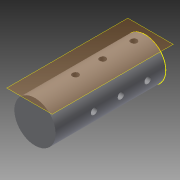
# Autodesk Inventor part: collector
Saved by Autodesk Inventor 2015 (Build 190159000, 159)
## iProperties
Created: 2014-11-05
Part Number: collector
Material: Generic
Document SubType Name: Modeling
Designer: lethcoec
Density: 1 g/cm^3
Appearance: Default
Author: lethcoec
Autodesk Inventor part; units mm, degrees
ref_plane "XY Plane" through (0, 0, 0) normal (0, 0, 1) x (1, 0, 0)
sketch "Sketch1" plane through (0, 0, 0) normal (0, 0, 1) x (1, 0, 0)
  circle A0 centre (0, 0) radius 19.05
  dimension "d0" = 38.1
  constraints: 1 centre point, 1 coincident
  measures "d0" diameter of A0
extrude "Extrusion1" add sketch "Sketch1" along normal blind 101.6
ref_plane "Work Plane1" through (19.05, 0, 0) normal (1, 0, 0) x (0, 1, 0)
sketch "Sketch3" plane through (19.05, 0, 0) normal (1, 0, 0) x (0, 1, 0)
  point P0 (0, 0)
sketch "Sketch4" plane through (19.05, 0, 0) normal (1, 0, 0) x (0, 1, 0)
  line L0 (0, 13.6144) -> (0, 19.5072)
  circle A0 centre (0, 16.5608) radius 2.9464
  point P0 (0, 0)
  dimension "d6" = 5.8928
  constraints: 2 end point, 1 midpoint, 1 vertical, 1 vertical alignment, 2 other
  measures "d6" distance of L0.start L0.end
hole "Hole1" at (19.05, 0, 16.5608) direction (-1, 0, 0) diameter 5.8928 end through all
sketch "Sketch5" plane through (19.05, 0, 0) normal (1, 0, 0) x (0, 1, 0)
  line L0 (0, 19.5072) -> (0, 38.354)
  line L1 (0, 38.354) -> (0, 44.2468)
  circle A0 centre (0, 41.3004) radius 2.9464
  point P0 (0, 0)
  dimension "d14" = 18.8468
  dimension "d15" = 5.8928
  constraints: 4 end point, 2 vertical, 1 midpoint, 1 vertical alignment, 2 other
  measures "d14" distance of L0.start L0.end
  measures "d15" distance of L0.end L1.end
hole "Hole2" at (19.05, 0, 41.3004) direction (-1, 0, 0) diameter 5.8928 end through all
sketch "Sketch6" plane through (19.05, 0, 0) normal (1, 0, 0) x (0, 1, 0)
  line L0 (0, 44.2467) -> (0, 63.0935)
  line L1 (0, 63.0935) -> (0, 68.9863)
  circle A0 centre (0, 66.0399) radius 2.9464
  point P0 (0, 0)
  dimension "d23" = 18.8468
  dimension "d24" = 5.8928
  constraints: 4 end point, 2 vertical, 1 midpoint, 1 vertical alignment, 2 other
  measures "d23" distance of L0.start L0.end
  measures "d24" distance of L0.end L1.end
hole "Hole3" at (19.05, 0, 66.0399) direction (-1, 0, 0) diameter 5.8928 end through all
sketch "Sketch7" plane through (0, 0, 0) normal (0, 0, -1) x (-1, 0, 0)
  circle A0 centre (0, 0) radius 19.05 projected
ref_plane "Work Plane2" through (0, 19.05, 0) normal (0, 1, 0) x (-1, 0, 0)
sketch "Sketch8" plane through (0, 19.05, 0) normal (0, 1, 0) x (-1, 0, 0)
  line L0 (0, 0) -> (0, 7.4041)
  line L1 (0, 7.4041) -> (0, 13.2969)
  circle A0 centre (0, 10.3505) radius 2.9464
  dimension "d33" = 7.4041
  dimension "d34" = 5.8928
  constraints: 4 end point, 2 vertical, 1 midpoint, 1 vertical alignment, 2 other
  measures "d33" distance of L0.start L0.end
  measures "d34" distance of L0.end L1.end
hole "Hole4" at (0, 19.05, 10.3505) direction (0, -1, 0) diameter 5.8928 end through all
sketch "Sketch9" plane through (0, 19.05, 0) normal (0, 1, 0) x (-1, 0, 0)
  line L0 (0, 13.2969) -> (0, 36.1569)
  line L1 (0, 36.1569) -> (0, 42.0497)
  circle A0 centre (0, 39.1033) radius 2.9464
  point P0 (0, 0)
  dimension "d42" = 22.86
  dimension "d43" = 5.8928
  constraints: 4 end point, 2 vertical, 1 midpoint, 1 vertical alignment, 2 other
  measures "d42" distance of L0.start L0.end
  measures "d43" distance of L0.end L1.end
sketch "Sketch10" plane through (0, 19.05, 0) normal (0, 1, 0) x (-1, 0, 0)
  line L0 (0, 42.0497) -> (0, 61.3283)
  line L1 (0, 61.3283) -> (0, 67.2211)
  circle A0 centre (0, 64.2747) radius 2.9464
  point P0 (0, 0)
  dimension "d44" = 19.2786
  dimension "d45" = 5.8928
  constraints: 4 end point, 2 vertical, 1 midpoint, 1 vertical alignment, 2 other
  measures "d44" distance of L0.start L0.end
  measures "d45" distance of L0.end L1.end
hole "Hole5" at (0, 19.05, 39.1033) direction (0, -1, 0) diameter 5.8928 end through all
hole "Hole6" at (0, 19.05, 64.2747) direction (0, -1, 0) diameter 5.8928 end through all
body "Solid1"
